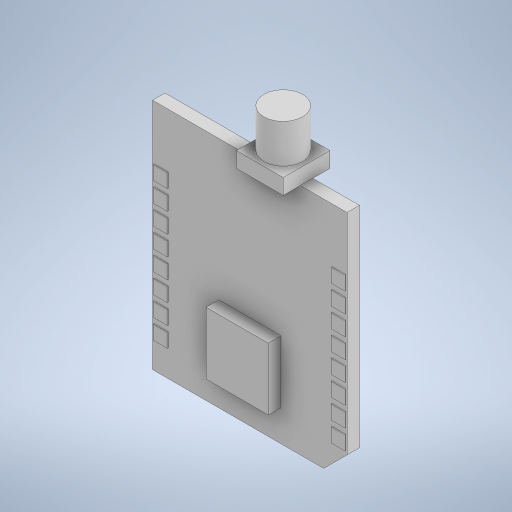
# Autodesk Inventor part: GNSS_board
Saved by Autodesk Inventor 2023 (Build 270158000, 158)
## iProperties
Created: 2023-03-23
Part Number: GNSS_board
Material: 一般
Document SubType Name: Modeling
Designer: 310611102
Density: 1 g/cm^3
Appearance: 預設
Author: 310611102
Autodesk Inventor part; units mm, degrees
ref_plane "YZ Plane" through (0, 0, 0) normal (1, 0, 0) x (0, 1, 0)
ref_plane "XZ Plane" through (0, 0, 0) normal (0, 1, 0) x (-1, 0, 0)
ref_plane "XY Plane" through (0, 0, 0) normal (0, 0, 1) x (1, 0, 0)
sketch "Sketch1" plane through (0, 0, 0) normal (0, 0, 1) x (1, 0, 0)
  line L0 (-12.5, 15) -> (12.5, 15)
  line L1 (12.5, 15) -> (12.5, -12)
  line L2 (9.5, -15) -> (-12.5, -15)
  line L3 (-12.5, -15) -> (-12.5, 15)
  line L4 (-12.5, 15) -> (12.5, -15) construction
  line L5 (12.5, 15) -> (-12.5, -15) construction
  line L6 (9.5, -15) -> (12.5, -12)
  point P0 (0, 0)
  dimension "d0" = 25
  dimension "d1" = 30
  dimension "d2" = 3
  dimension "d3" = 3
  constraints: 14 end point, 2 midpoint, 2 parallel, 2 point on line, 1 horizontal, 1 perpendicular
  measures "d0" distance of L0.start L0.end
  measures "d1" distance of L2.end L0.start
  measures "d2" distance of L2.start L4.end
  measures "d3" distance of L1.end L4.end
extrude "Extrusion1" add sketch "Sketch1" along normal blind 1.6
sketch "Sketch2" plane through (0, 0, 1.6) normal (0, 0, 1) x (1, 0, 0)
  line L0 (-4, -3) -> (4, -3)
  line L1 (4, -3) -> (4, -11)
  line L2 (4, -11) -> (-4, -11)
  line L3 (-4, -11) -> (-4, -3)
  line L4 (-4, -3) -> (4, -11) construction
  line L5 (4, -3) -> (-4, -11) construction
  line L6 (-12.5, -15) -> (9.5, -15) projected
  point P0 (0, 0)
  point P1 (0, -7)
  dimension "d6" = 8
  dimension "d7" = 8
  dimension "d8" = 8
  constraints: 12 end point, 2 midpoint, 2 parallel, 1 horizontal, 1 perpendicular
  measures "d6" distance of L0.start L0.end
  measures "d7" distance of L0.end L1.end
  measures "d8" distance from line of L6 point (0, -7)
extrude "Extrusion2" add sketch "Sketch2" along normal blind 1.6
sketch "Sketch5" plane through (0, 0, 1.6) normal (0, 0, 1) x (1, 0, 0)
  line L0 (-12.3, 8) -> (-10.5, 8)
  line L1 (-10.5, 8) -> (-10.5, 6.2)
  line L2 (-10.5, 6.2) -> (-12.3, 6.2)
  line L3 (-12.3, 6.2) -> (-12.3, 8)
  line L4 (-12.3, 8) -> (-10.5, 6.2) construction
  line L5 (-10.5, 8) -> (-12.3, 6.2) construction
  line L6 (-12.5, 15) -> (-12.5, -15) projected
  line L7 (-12.3, 3.66) -> (-12.3, 5.46)
  line L8 (-12.3, 5.46) -> (-10.5, 5.46)
  line L9 (-10.5, 5.46) -> (-10.5, 3.66)
  line L10 (-10.5, 3.66) -> (-12.3, 3.66)
  line L11 (-12.3, 1.12) -> (-12.3, 2.92)
  line L12 (-12.3, 2.92) -> (-10.5, 2.92)
  line L13 (-10.5, 2.92) -> (-10.5, 1.12)
  line L14 (-10.5, 1.12) -> (-12.3, 1.12)
  line L15 (-12.3, -1.42) -> (-12.3, 0.38)
  line L16 (-12.3, 0.38) -> (-10.5, 0.38)
  line L17 (-10.5, 0.38) -> (-10.5, -1.42)
  line L18 (-10.5, -1.42) -> (-12.3, -1.42)
  line L19 (-12.3, -3.96) -> (-12.3, -2.16)
  line L20 (-12.3, -2.16) -> (-10.5, -2.16)
  line L21 (-10.5, -2.16) -> (-10.5, -3.96)
  line L22 (-10.5, -3.96) -> (-12.3, -3.96)
  line L23 (-12.3, -6.5) -> (-12.3, -4.7)
  line L24 (-12.3, -4.7) -> (-10.5, -4.7)
  line L25 (-10.5, -4.7) -> (-10.5, -6.5)
  line L26 (-10.5, -6.5) -> (-12.3, -6.5)
  line L27 (-12.3, -9.04) -> (-12.3, -7.24)
  line L28 (-12.3, -7.24) -> (-10.5, -7.24)
  line L29 (-10.5, -7.24) -> (-10.5, -9.04)
  line L30 (-10.5, -9.04) -> (-12.3, -9.04)
  line L31 (-12.3, -11.58) -> (-12.3, -9.78)
  line L32 (-12.3, -9.78) -> (-10.5, -9.78)
  line L33 (-10.5, -9.78) -> (-10.5, -11.58)
  line L34 (-10.5, -11.58) -> (-12.3, -11.58)
  line L35 (12.5, 15) -> (-12.5, 15) projected
  line L36 (10.56, 6.2) -> (10.56, 8)
  line L37 (10.56, 8) -> (12.36, 8)
  line L38 (12.36, 8) -> (12.36, 6.2)
  line L39 (12.36, 6.2) -> (10.56, 6.2)
  line L40 (10.56, 3.66) -> (10.56, 5.46)
  line L41 (10.56, 5.46) -> (12.36, 5.46)
  line L42 (12.36, 5.46) -> (12.36, 3.66)
  line L43 (12.36, 3.66) -> (10.56, 3.66)
  line L44 (10.56, 1.12) -> (10.56, 2.92)
  line L45 (10.56, 2.92) -> (12.36, 2.92)
  line L46 (12.36, 2.92) -> (12.36, 1.12)
  line L47 (12.36, 1.12) -> (10.56, 1.12)
  line L48 (10.56, -1.42) -> (10.56, 0.38)
  line L49 (10.56, 0.38) -> (12.36, 0.38)
  line L50 (12.36, 0.38) -> (12.36, -1.42)
  line L51 (12.36, -1.42) -> (10.56, -1.42)
  line L52 (10.56, -3.96) -> (10.56, -2.16)
  line L53 (10.56, -2.16) -> (12.36, -2.16)
  line L54 (12.36, -2.16) -> (12.36, -3.96)
  line L55 (12.36, -3.96) -> (10.56, -3.96)
  line L56 (10.56, -6.5) -> (10.56, -4.7)
  line L57 (10.56, -4.7) -> (12.36, -4.7)
  line L58 (12.36, -4.7) -> (12.36, -6.5)
  line L59 (12.36, -6.5) -> (10.56, -6.5)
  line L60 (10.56, -9.04) -> (10.56, -7.24)
  line L61 (10.56, -7.24) -> (12.36, -7.24)
  line L62 (12.36, -7.24) -> (12.36, -9.04)
  line L63 (12.36, -9.04) -> (10.56, -9.04)
  line L64 (10.56, -11.58) -> (10.56, -9.78)
  line L65 (10.56, -9.78) -> (12.36, -9.78)
  line L66 (12.36, -9.78) -> (12.36, -11.58)
  line L67 (12.36, -11.58) -> (10.56, -11.58)
  point P0 (0, 0)
  point P1 (-11.4, 7.1)
  point P2 (2, 15)
  dimension "d19" = 1.8
  dimension "d20" = 1.8
  dimension "d21" = 1.1
  dimension "d24" = 2.54
  dimension "d29" = 7
  dimension "d32" = 22.86
  constraints: 132 end point, 2 collinear, 2 horizontal, 2 midpoint, 2 parallel, 1 perpendicular, 1 vertical, 118 other
  measures "d19" distance of L0.start L0.end
  measures "d20" distance of L2.end L0.start
  measures "d21" distance from line of L6 point (-11.4, 7.1)
  measures "d24" distance of L2.end L7.start
  measures "d29" distance between parallel lines of L35 L0
  measures "d32" distance of L2.end L36.start
extrude "Extrusion5" add sketch "Sketch5" along normal blind 0.1
sketch "Sketch6" plane through (-12.5, 15, 0) normal (0, 1, 0) x (1, 0, 0)
  line L0 (19, -3.8) -> (13, -3.8)
  line L1 (13, -3.8) -> (13, 2.2)
  line L2 (13, 2.2) -> (19, 2.2)
  line L3 (19, 2.2) -> (19, -3.8)
  line L4 (19, -3.8) -> (13, 2.2) construction
  line L5 (13, -3.8) -> (19, 2.2) construction
  line L6 (25, 0) -> (25, -1.6) projected
  point P0 (12.5, 0)
  point P1 (16, -0.8)
  point P2 (25, -0.8)
  dimension "d39" = 6
  dimension "d40" = 6
  dimension "d41" = 6
  constraints: 12 end point, 3 midpoint, 2 parallel, 1 horizontal, 1 horizontal alignment, 1 perpendicular
  measures "d39" distance of L0.end L1.end
  measures "d40" distance of L0.start L0.end
  measures "d41" distance between parallel lines of L6 L3
extrude "Extrusion6" add sketch "Sketch6" along normal blind 2
sketch "Sketch7" plane through (-12.5, 17, 0) normal (0, 1, 0) x (1, 0, 0)
  circle A0 centre (16, -0.8) radius 2.5
  line L0 (13, -3.8) -> (19, -3.8) projected
  line L1 (13, 2.2) -> (13, -3.8) projected
  point P0 (12.5, 0)
  point P1 (16, -3.8)
  point P2 (13, -0.8)
  dimension "d44" = 5
  constraints: 2 midpoint, 1 centre point, 1 horizontal alignment, 1 vertical alignment
  measures "d44" diameter of A0
extrude "Extrusion7" add sketch "Sketch7" along normal blind 5
equation "\"d3\" = d2"
body "Solid1"
